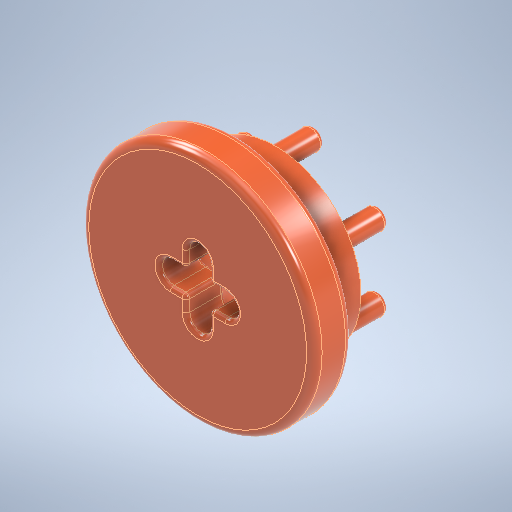
# Autodesk Inventor part: Steering Gear Plate
Saved by Autodesk Inventor 2025.2 (Build 292293000, 293)
## iProperties
Created: 2025-02-06
Part Number: Steering Gear Plate
Material: Generic
Document SubType Name: Modeling
Designer: eason
Density: 1 g/cm^3
Appearance: Smooth - Light Orange
Author: eason
Autodesk Inventor part; units mm, degrees
ref_plane "YZ Plane" through (0, 0, 0) normal (1, 0, 0) x (0, 1, 0)
ref_plane "XZ Plane" through (0, 0, 0) normal (0, 1, 0) x (-1, 0, 0)
ref_plane "XY Plane" through (0, 0, 0) normal (0, 0, 1) x (1, 0, 0)
sketch "Sketch1" plane through (0, 0, 0) normal (0, 0, 1) x (1, 0, 0)
  circle A0 centre (0, 0) radius 15
  circle A1 centre (0, 0) radius 2
  circle A2 centre (0, 0) radius 5
  circle A3 centre (3.5, 0) radius 1.5
  circle A4 centre (-3.5, 0) radius 1.5
  line L0 (-21, 0) -> (21, 0) projected
  circle A5 centre (0, 3.5) radius 1.5
  circle A6 centre (0, -3.5) radius 1.5
  line L1 (0, -21) -> (0, 21) projected
  line L2 (-1.5, -3.5) -> (-1.5, -2)
  line L3 (-3.5, -1.5) -> (-2, -1.5)
  arc A7 (-1.5, -2) -> (-2, -1.5) centre (-2, -2) ccw
  line L4 (1.5, -3.5) -> (1.5, -2)
  arc A8 (2, -1.5) -> (1.5, -2) centre (2, -2) ccw
  line L5 (3.5, -1.5) -> (2, -1.5)
  line L6 (3.5, 1.5) -> (2, 1.5)
  arc A9 (1.5, 2) -> (2, 1.5) centre (2, 2) ccw
  line L7 (1.5, 3.5) -> (1.5, 2)
  line L8 (-1.5, 3.5) -> (-1.5, 2)
  arc A10 (-2, 1.5) -> (-1.5, 2) centre (-2, 2) ccw
  line L9 (-3.5, 1.5) -> (-2, 1.5)
  point P0 (-5, 0)
  point P1 (-2, 0)
  point P2 (2, 0)
  point P3 (5, 0)
  point P4 (0, -5)
  point P5 (0, -2)
  point P6 (0, 2)
  point P7 (0, 5)
  point P8 (1.5, 3.5)
  point P9 (1.5, -3.5)
  dimension "d0" = 30
  dimension "d2" = 10
  dimension "d60" = 3
  dimension "d61" = 0.5
  dimension "d64" = 360
  constraints: 16 end point, 9 centre point, 8 point on circle, 6 tangent, 4 point on line, 3 coincident, 2 horizontal, 2 vertical, 43 other
  measures "d0" diameter of A0
  measures "d2" diameter of A2
  measures "d60" radial gap between concentric circles of A2 A1
  measures "d61" radius of A7
extrude "Extrusion1" add sketch "Sketch1" along normal blind 5 contours L0 A2 L1 A0 | A0 L1 A2 L0 | L1 A2 L0 A0 | A0 L0 A2 L1 | A3 L6 A9 L7 A5 A2 | A2 A6 L4 A8 L5 A3 | A5 L8 A10 L9 A4 A2 | A2 A4 L3 A7 L2 A6
ref_plane "Work Plane1" through (0, 0, 2.5) normal (0, 0, 1) x (1, 0, 0)
sketch "Sketch5" plane through (0, 0, 0) normal (0, 0, -1) x (-1, 0, 0)
  line L0 (0, 0) -> (-5.2212, -14.062) construction
  circle A0 centre (0, 0) radius 15 projected
  line L1 (0, -21) -> (0, 21) projected
  circle A1 centre (-4.351, -11.7183) radius 2.5
  arc A2 (0.0912, -10.9996) -> (-7.2478, -8.2746) centre (-4.351, -11.7183) ccw
  arc A3 (0.0912, -10.9996) -> (-7.2478, -8.2746) centre (0, 0) ccw
  circle A4 centre (0, 0) radius 8
  point P0 (-2.7846, -7.4997)
  dimension "d25" = 20.37
  dimension "d26" = 5
  dimension "d30" = 2
  dimension "d32" = 4
  constraints: 4 centre point, 4 point on circle, 3 coincident, 2 end point, 1 point on line, 1 tangent, 3 other
  measures "d25" angle of L1 L0
  measures "d26" diameter of A1
  measures "d30" radial gap between concentric circles of A2 A1
extrude "Extrusion5" add sketch "Sketch5" along normal blind 5 contours A1 | A3 A2 L1 A4 | L1 A4 A2 A3 | A2 A4 L1
sketch "Sketch8" plane through (0, 0, -5) normal (0, 0, -1) x (-1, 0, 0)
  circle A0 centre (0, 9.5) radius 1.5 construction
  circle A1 centre (0, 0) radius 8 projected
  arc A2 (0.0912, -10.9996) -> (-7.2478, -8.2746) centre (0, 0) ccw projected
  line L0 (0, -21) -> (0, 21) projected
  circle A3 centre (0, 9.5) radius 1.3
  circle A4 centre (-8.2272, 4.75) radius 1.3
  circle A5 centre (-8.2272, -4.75) radius 1.3
  circle A6 centre (0, -9.5) radius 1.3
  circle A7 centre (8.2272, -4.75) radius 1.3
  circle A8 centre (8.2272, 4.75) radius 1.3
  point P0 (-2.7846, -7.4997)
  dimension "d70" = 0.2
  dimension "d73" = 360
  constraints: 7 centre point, 1 coincident, 1 point on line, 1 tangent, 15 other
  measures "d70" radial gap between concentric circles of A3 A0
extrude "Extrusion8" add sketch "Sketch8" along normal blind 5 contours A3 L0 | L0 A3 | A4 | A5 | A7 | A8
fillet "Fillet5" radius 1 4 edges at (-15, 0, 5) (-12.315, 8.5639, 0) (12.315, -8.5639, 0) (6.851, -11.7183, -5)
fillet "Fillet6" radius 0.5 5 edges at (1.3, 9.5, -10) (-6.9272, 4.75, -10) (-6.9272, -4.75, -10) (9.5272, -4.75, -10) (9.5272, 4.75, -10)
fillet "Fillet7" radius 0.5 32 edges at (-5, 0, 5) (-2.75, 1.5, 5) (-1.6464, 1.6464, 5) (-1.5, 2.75, 5) (0, 5, 5) (1.5, 2.75, 5) (1.6464, 1.6464, 5) (2.75, 1.5, 5) (5, 0, 5) (2.75, -1.5, 5) (1.6464, -1.6464, 5) (1.5, -2.75, 5) (0, -5, 5) (-1.5, -2.75, 5) (-1.6464, -1.6464, 5) (-2.75, -1.5, 5) (1.5, -2.75, 0) (0, -5, 0) (-1.5, -2.75, 0) (-1.6464, -1.6464, 0) (-2.75, -1.5, 0) (-5, 0, 0) (-2.75, 1.5, 0) (-1.6464, 1.6464, 0) (-1.5, 2.75, 0) (0, 5, 0) (1.5, 2.75, 0) (1.6464, 1.6464, 0) (2.75, 1.5, 0) (5, 0, 0) (2.75, -1.5, 0) (1.6464, -1.6464, 0)
body "Solid1"
